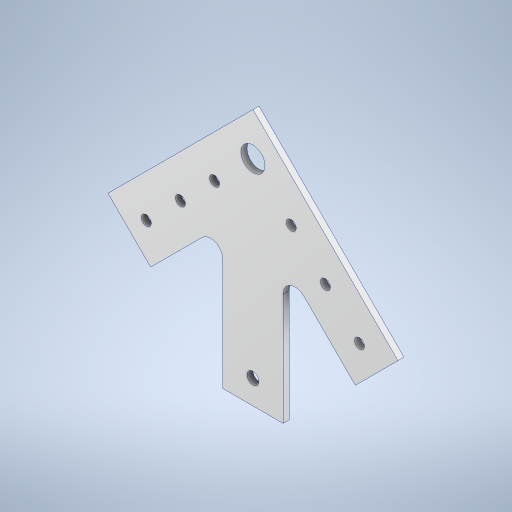
# Autodesk Inventor part: CH-1-HipPivotPlate
Saved by Autodesk Inventor 2023 (Build 270158000, 158)
## iProperties
Created: 2023-03-14
Part Number: CH-1-HipPivotPlate
Material: Aluminum 6061
Document SubType Name: Modeling
Designer: megan
Density: 2.7 g/cm^3
Appearance: Aluminum - Flat
Author: megan
Autodesk Inventor part; units mm, degrees
ref_plane "YZ Plane" through (0, 0, 0) normal (1, 0, 0) x (0, 1, 0)
ref_plane "XZ Plane" through (0, 0, 0) normal (0, 1, 0) x (-1, 0, 0)
ref_plane "XY Plane" through (0, 0, 0) normal (0, 0, 1) x (1, 0, 0)
sketch "Sketch1" plane through (0, 0, 0) normal (0, 0, 1) x (1, 0, 0)
  line L0 (-53.8815, -76.3322) -> (-15.875, -38.3256)
  line L1 (-53.8815, -76.3322) -> (-76.3322, -53.8815)
  line L2 (-76.3322, -53.8815) -> (0, 22.4506)
  line L3 (53.8815, -76.3322) -> (15.875, -38.3256)
  line L4 (53.8815, -76.3322) -> (76.3322, -53.8815)
  line L5 (76.3322, -53.8815) -> (0, 22.4506)
  line L6 (-106.865, 0) -> (106.865, 0) projected
  line L7 (-15.875, -38.3256) -> (-15.875, -112.7)
  line L8 (-15.875, -112.7) -> (15.875, -112.7)
  line L9 (15.875, -112.7) -> (15.875, -38.3256)
  circle A0 centre (0, -100) radius 3.175
  line L10 (0, -139.7301) -> (0, 49.4808) projected
  circle A1 centre (0, 0) radius 6.35
  point P0 (0, -112.7)
  dimension "d13" = 31.75
  dimension "d38" = 100
  dimension "d39" = 45
  dimension "d41" = 15.875
  dimension "d43" = 112.7
  dimension "d44" = 12.7
  dimension "d47" = 15.875
  dimension "d48" = 76.2
  constraints: 18 end point, 4 perpendicular, 3 equal length, 3 parallel, 2 centre point, 1 coincident, 1 midpoint, 1 point on line
  measures "d13" distance of L0.start L1.end
  measures "d38" distance of point (0, 0) A0.centre
  measures "d39" angle of L7 L0
  measures "d41" distance between parallel lines of L7 L10
  measures "d43" distance between parallel lines of L6 L8
  measures "d44" diameter of A1
  measures "d47" distance from line of L3 point (0, 0)
  measures "d48" distance between parallel lines of L3 L1
extrude "Extrusion1" add sketch "Sketch1" along normal blind 3.175 contours L1 L2 L6 A1 L10 A0 L8 L7 L0 | L2 L10 A1 L6 | L10 A0 A1 L6 L5 L4 L3 L9 L8 | L5 L6 A1 L10
sketch "Sketch2" plane through (0, 0, 3.175) normal (0, 0, 1) x (1, 0, 0)
  line L0 (-76.3322, -53.8815) -> (-53.8815, -76.3322) projected
  line L1 (-65.1069, -65.1069) -> (14.4203, 14.4203)
  line L2 (53.8815, -76.3322) -> (76.3322, -53.8815) projected
  line L3 (76.3322, -53.8815) -> (0, 22.4506) projected
  line L4 (0, 22.4506) -> (-76.3322, -53.8815) projected
  line L5 (-76.3322, -53.8815) -> (-53.8815, -76.3322) projected
  line L6 (-53.8815, -76.3322) -> (-15.875, -38.3256) projected
  line L7 (15.875, -38.3256) -> (53.8815, -76.3322) projected
  circle A0 centre (-56.1266, -56.1266) radius 2.65
  circle A1 centre (-38.1661, -38.1661) radius 2.65
  circle A2 centre (-20.2056, -20.2056) radius 2.65
  line L8 (-15.875, -38.3256) -> (-15.875, -112.7) projected
  line L9 (-15.875, -112.7) -> (15.875, -112.7) projected
  line L10 (15.875, -112.7) -> (15.875, -38.3256) projected
  point P0 (0, 0)
  dimension "d17" = 5.3
  dimension "d18" = 12.7
  dimension "d21" = 25.4
  constraints: 3 centre point, 2 end point, 1 midpoint, 1 perpendicular, 1 point on line, 5 other
  measures "d17" diameter of A0
  measures "d18" distance from line of A0.centre L0
  measures "d21" distance of A0.centre A1.centre
extrude "Extrusion2" cut sketch "Sketch2" against normal blind 3.175 contours A0 L1 | L1 A0 | A2 L1 | L1 A2 | A1 L1 | L1 A1
mirror "Mirror1" about plane through (0, 0, 0) normal (1, 0, 0) of "Extrusion2"
fillet "Fillet3" radius 6.35 2 edges at (-15.875, -38.3256, 1.5875) (15.875, -38.3256, 1.5875)
equation "\"d41\" = 0.5 * d13"
equation "\"d47\" = d41"
equation "\"d15\" = plateThickness"
equation "\"d17\" = boltDiameter"
equation "\"d26\" = plateThickness"
equation "\"topDiameter\" = 25"
equation "\"shaftLength\" = 76.2"
equation "\"bearingDiameter\" = 28.62"
equation "\"plateThickness\" = 3.175"
equation "\"theta12\" = 100deg"
equation "\"boltDiameter\" = 5.3"
equation "\"gearboxLength\" = 101.6"
equation "\"boltedLength\" = 76.2"
equation "\"innerBoltSpacing\" = 12.7"
equation "\"outerBoltSpacing\" = 12.7"
body "Solid1"
